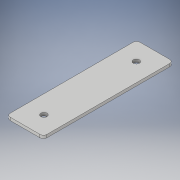
# Autodesk Inventor part: HOVER-plate-b
Saved by Autodesk Inventor 2019.4 (Build 234330000, 330)
## iProperties
Created: 2020-04-17
Part Number: HOVER-plate-b
Material: Generic
Document SubType Name: Sheet Metal
Designer: Phil
Density: 1 g/cm^3
Sheet Metal Rule: Default
Appearance: Default
Flat Pattern Width: 3.81 cm
Flat Pattern Length: 13.4874 cm
Flat Pattern Area: 51.387 cm^2
Sheet Metal Width: 1.500 in
Sheet Metal Length: 5.310 in
Sheet Metal Area: 7.965 in^2
Author: Phil
Autodesk Inventor part; units mm, degrees
ref_plane "YZ Plane" through (0, 0, 0) normal (1, 0, 0) x (0, 1, 0)
ref_plane "XZ Plane" through (0, 0, 0) normal (0, 1, 0) x (-1, 0, 0)
ref_plane "XY Plane" through (0, 0, 0) normal (0, 0, 1) x (1, 0, 0)
sketch "Sketch1" plane through (0, 0, 0) normal (0, 1, 0) x (-1, 0, 0)
  line L0 (-15.494, -67.437) -> (15.494, -67.437)
  line L1 (19.05, -63.881) -> (19.05, 63.881)
  line L2 (15.494, 67.437) -> (-15.494, 67.437)
  line L3 (-19.05, 63.881) -> (-19.05, -63.881)
  line L4 (-19.05, -67.437) -> (19.05, 67.437) construction
  line L5 (19.05, -67.437) -> (-19.05, 67.437) construction
  circle A0 centre (0, 47.879) radius 3.175
  circle A1 centre (0, -48.133) radius 3.175
  arc A2 (19.05, 63.881) -> (15.494, 67.437) centre (15.494, 63.881) ccw
  arc A3 (-15.494, 67.437) -> (-19.05, 63.881) centre (-15.494, 63.881) ccw
  arc A4 (15.494, -67.437) -> (19.05, -63.881) centre (15.494, -63.881) ccw
  arc A5 (-19.05, -63.881) -> (-15.494, -67.437) centre (-15.494, -63.881) ccw
  point P0 (0, 0)
  dimension "d0" = 38.1
  dimension "d1" = 134.874
  dimension "d2" = 6.35
  dimension "d3" = 19.558
  dimension "d4" = 6.35
  dimension "d5" = 96.012
  dimension "d6" = 3.556
  measures "d0" distance of L5.end L4.end
  measures "d1" distance of L4.end L5.start
  measures "d2" diameter of A0
  measures "d3" distance from line of A0.centre L2
  measures "d4" diameter of A1
  measures "d5" distance of A1.centre A0.centre
  measures "d6" radius of A2
extrude "Plate1" add sketch "Sketch1" along normal blind 3.048
equation "\"d7\" = Thickness"
equation "\"BendRadius\" = Thickness"
equation "\"BendReliefWidth\" = Thickness"
equation "\"BendReliefDepth\" = 0.5 * Thickness"
equation "\"CornerReliefSize\" = 4 * Thickness"
equation "\"MinimumRemnant\" = 2 * Thickness"
equation "\"TransitionRadius\" = BendRadius"
equation "\"JacobiRadiusSize\" = BendRadius"
equation "\"GapSize\" = Thickness"
equation "\"Thickness\" = 3.048"
body "Solid1"
